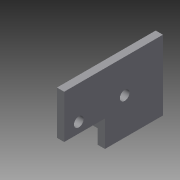
# Autodesk Inventor part: bart y endstop v2
Saved by Autodesk Inventor 2014 SP1 (Build 180222100, 222)
## iProperties
Created: 2015-06-04
Part Number: bart y endstop v2
Material: Generic
Document SubType Name: Modeling
Designer: Mon
Density: 1 g/cm^3
Appearance: Default
Author: Mon
Autodesk Inventor part; units mm, degrees
ref_plane "YZ Plane" through (0, 0, 0) normal (1, 0, 0) x (0, 1, 0)
ref_plane "XZ Plane" through (0, 0, 0) normal (0, 1, 0) x (-1, 0, 0)
ref_plane "XY Plane" through (0, 0, 0) normal (0, 0, 1) x (1, 0, 0)
sketch "Sketch1" plane through (0, 0, 0) normal (0, 0, 1) x (1, 0, 0)
  line L0 (0, 0) -> (16.5, 0)
  line L1 (16.5, 0) -> (16.5, -24)
  line L2 (16.5, -24) -> (0, -24)
  line L3 (0, -24) -> (0, 0)
  line L4 (24.2611, -12.002) -> (-7.0214, -12.002)
  line L5 (10.5138, 0) -> (10.5138, -25.2396)
  line L6 (10.5138, -12.002) -> (10.5138, -20.002) construction
  line L7 (10.5138, -12.002) -> (10.5138, -4.002) construction
  circle A0 centre (10.5138, -4.002) radius 2
  circle A1 centre (10.5138, -20.002) radius 2
  circle A2 centre (4.1138, -12.002) radius 2
  dimension "d0" = 16.5
  dimension "d1" = 24
  dimension "d2" = 8
  dimension "d3" = 8
  dimension "d4" = 4
  dimension "d5" = 4
  dimension "d7" = 4
  constraints: 16 end point, 4 point on line, 3 centre point, 3 perpendicular, 2 coincident, 2 collinear, 2 parallel, 1 horizontal
  measures "d0" distance of L1.end L2.end
  measures "d1" distance of L0.end L1.end
  measures "d2" distance of L6.start L6.end
  measures "d3" distance of L6.start L7.end
  measures "d4" diameter of A0
  measures "d5" diameter of A1
  measures "d7" diameter of A2
extrude "Extrusion1" add sketch "Sketch1" along normal blind 3 contours L0 L5 A0 L4 A2 L3 | L0 L1 L4 L5 A0 | L4 A2 L5 A1 L2 L3 | L1 L2 L5 A1 L4
sketch "Sketch2" plane through (16.5, -24, 0) normal (1, 0, 0) x (0, 0, -1)
  line L0 (-3, -16.8669) -> (-3, 24)
  line L1 (-3, -16.8669) -> (-23, -16.8669)
  line L2 (-23, -16.8669) -> (5.9335, -16.8669)
  line L3 (5.9335, -16.8669) -> (5.9335, 24)
  line L4 (5.9335, 24) -> (-23, 24)
  line L5 (-23, 24) -> (-23, -16.8669)
  circle A0 centre (-9.1835, 8.1747) radius 2
  line L6 (-9.1835, 8.1747) -> (-9.1835, -10.8253) construction
  circle A1 centre (-9.1835, -10.8253) radius 2
  dimension "d11" = 20
  dimension "d12" = 4
  dimension "d13" = 19
  dimension "d14" = 4
  constraints: 14 end point, 4 parallel, 2 centre point, 2 perpendicular, 1 coincident, 1 horizontal
  measures "d11" distance of L0.start L1.end
  measures "d12" diameter of A0
  measures "d13" distance of L6.start L6.end
  measures "d14" diameter of A1
extrude "Extrusion2" add sketch "Sketch2" along normal blind 3
sketch "Sketch3" plane through (16.5, -24, 0) normal (-1, 0, 0) x (0, 0, 1)
  line L0 (-5.9335, -16.8669) -> (-5.9335, 24) projected
  line L1 (-5.9335, 0.0047) -> (4.9967, 0.0047)
  line L2 (4.9967, 0.0047) -> (4.9967, -16.8669)
  line L3 (4.9967, -16.8669) -> (-5.9335, -16.8669)
  line L4 (-5.9335, -16.8669) -> (-5.9335, 0.0047)
  constraints: 8 end point, 2 parallel, 1 horizontal, 1 perpendicular, 1 point on line
extrude "Extrusion3" cut sketch "Sketch3" against normal through all
body "Solid1"
